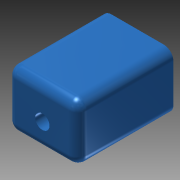
# Autodesk Inventor part: PanelLedge
Saved by Autodesk Inventor 2016 (Build 200138000, 138)
## iProperties
Category: Print
Created: 2015-03-13
Part Number: PanelLedge
Material: ABS Plastic
Document SubType Name: Modeling
Designer: Jack
Density: 1.06 g/cm^3
Appearance: Cyan
Mass: 2.95082 g
Surface Area: 16.5334 cm^2
Volume: 2.7838 cm^3
Author: Jack
Title: Panel Ledge
Autodesk Inventor part; units mm, degrees
ref_plane "YZ Plane" through (0, 0, 0) normal (1, 0, 0) x (0, 1, 0)
ref_plane "XZ Plane" through (0, 0, 0) normal (0, 1, 0) x (-1, 0, 0)
ref_plane "XY Plane" through (0, 0, 0) normal (0, 0, 1) x (1, 0, 0)
sketch "Sketch1" plane through (0, 0, 0) normal (0, 0, 1) x (1, 0, 0)
  line L0 (0, 0) -> (15, 0)
  line L1 (15, 0) -> (15, 20)
  line L2 (15, 20) -> (0, 20)
  line L3 (0, 20) -> (0, 0)
  dimension "d0" = 15
  dimension "d1" = 20
  constraints: 8 end point, 2 parallel, 1 horizontal, 1 perpendicular
  measures "d0" distance of L2.end L1.end
  measures "d1" distance of L0.end L1.end
extrude "Extrusion1" add sketch "Sketch1" along normal blind 12
sketch "Sketch5" plane through (0, 0, 0) normal (0, 0, -1) x (-1, 0, 0)
  line L0 (0, 20) -> (0, 0) projected
  line L1 (-15, 20) -> (0, 20) projected
  line L2 (-11.5, 16) -> (-3.5, 16)
  line L3 (-3.5, 16) -> (-3.5, 7.5)
  line L4 (-3.5, 7.5) -> (-11.5, 7.5)
  line L5 (-11.5, 7.5) -> (-11.5, 16)
  dimension "d15" = 8
  dimension "d16" = 8.5
  dimension "d17" = 4
  dimension "d18" = 3.5
  constraints: 8 end point, 2 parallel, 1 horizontal, 1 perpendicular
  measures "d15" distance of L3.end L4.end
  measures "d16" distance of L2.end L3.end
  measures "d17" distance between parallel lines of L1 L2
  measures "d18" distance between parallel lines of L0 L3
extrude "Extrusion4" cut sketch "Sketch5" against normal blind 9.237
fillet "Fillet1" radius 4 2 edges at (11.5, 11.75, 9.237) (3.5, 11.75, 9.237)
sketch "Sketch6" plane through (3.5, 16, 0) normal (0, -1, 0) x (1, 0, 0)
  arc A0 (8, 5.237) -> (0, 5.237) centre (4, 5.237) ccw projected
  circle A1 centre (4, 5.237) radius 2
  point P0 (-3.5, 0)
  dimension "d22" = 4
  constraints: 1 centre point, 1 coincident
  measures "d22" diameter of A1
extrude "Extrusion5" cut sketch "Sketch6" against normal up to surface (4 mm away)
chamfer "Chamfer1" distance 2 angle 45 1 edges at (5.5, 16, 5.237)
sketch "Sketch7" plane through (3.5, 7.5, 0) normal (0, 1, 0) x (1, 0, 0)
  arc A0 (0, -5.237) -> (8, -5.237) centre (4, -5.237) ccw projected
  circle A1 centre (4, -5.237) radius 1.5
  point P0 (-3.5, 0)
  dimension "d28" = 3
  constraints: 1 centre point, 1 coincident
  measures "d28" diameter of A1
extrude "Extrusion6" cut sketch "Sketch7" against normal up to surface (7.5 mm away)
fillet "Fillet2" radius 2 8 edges at (15, 0, 6) (0, 0, 6) (15, 10, 0) (15, 10, 12) (0, 10, 0) (7.5, 0, 0) (7.5, 0, 12) (0, 10, 12)
body "Solid1"
